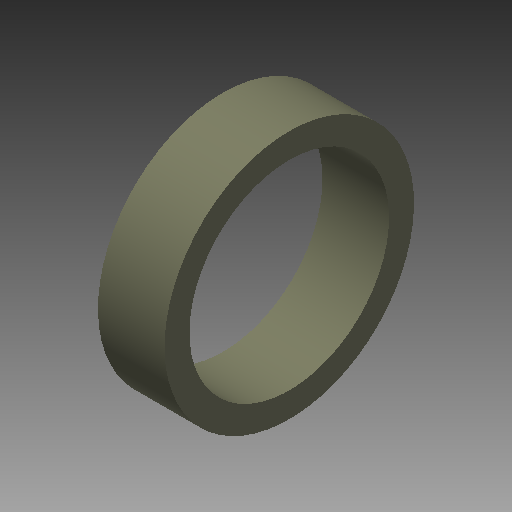
# Autodesk Inventor part: UMHSL30_k
Saved by Autodesk Inventor 2019 (Build 230136000, 136)
## iProperties
Category: PARTsolutions
Company: MISUMI
Created: 2015-12-01
Part Number: UMHSL30_k
Catalog Web Link: www.cadenas.de
Description: UMHSH, UMHS, UMHSL ,UMHAH, UMHA, UMHAL_k-Urethane Rollers - Set Screw Type
Vendor: MISUMI
Document SubType Name: Modeling
Designer: psAdmin
Manufacturer: MISUMI
Mass: 2.03575 g
Surface Area: 18.6611 cm^2
Volume: 2.03575 cm^3
Density: 1 g/cm^3
Material: Generic
Appearance: PSOLRGB-252-255-188
PSOL_IDENT_0: {$CADENAS_DATA\23d-libs\misumi\metric\53_rollers\umhsh\umhsh_k.prj},201 {VTYP=3D},{NB=UMHSL30_k},{LI
PSOL_IDENT_1: NA=UMHSL30},{NN=UMHSH, UMHS, UMHSL ,UMHAH, UMHA, UMHAL_k},{DATE=06.11.2015 05:15:16},{GEOMDATE=30.10
PSOL_IDENT_2: .2015 01:03:12},{VERSION=},{LINEID=70},{LINESUBID=-1},{WBVAR=MATC,HARD}  {NB=UMHSL30_k},{LINA=UMHSL3
PSOL_IDENT_3: 0},{KT=DUMMY},{PN=UMHSL30},{TYPE=UMHSL},{MATC=1},{MATCALG= '1','304 Stainless Steel','2','5052 Alumi
PSOL_IDENT_4: num Alloy'},{MATU=Urethane (Natural Color)},{HARD=A50},{COLOR=0.99,1.00,0.74,0.00},{NO=30},{D=30},{D
PSOL_IDENT_5: D=6},{D1=16},{D2=24},{D2X=24},{W=8},{L=20},{R=6.0},{M=3}
NN: UMHSH, UMHS, UMHSL ,UMHAH, UMHA, UMHAL_k
NT: Urethane Rollers - Set Screw Type
NB: UMHSL30_k
NBSYN: $PN._k
LINA: UMHSL30
PN: UMHSL30
MATC: 304 Stainless Steel
MATU: Urethane (Natural Color)
HARD: Shore A50
NO: 30
D: 30
DD: 6
D1: 16
D2: 24
W: 8
L: 20
M: 3
SUPPLIER: MISUMI
ARTICLENO: UMHSL30_k
BOMINFO: UMHSL30
CREATOR: CADENAS GmbH
Title: UMHSL30
Author: Cadenas PARTsolutions
Comments: Urethane Rollers - Set Screw Type
Autodesk Inventor part; units mm, degrees
sketch "Sketch_1" plane through (0, 0, 0) normal (0, 0, 1) x (1, 0, 0)
  line L0 (4, 0) -> (-4, 0)
  line L1 (-4, 15) -> (-4, 12)
  line L2 (-4, 12) -> (4, 12)
  line L3 (4, 12) -> (4, 15)
  line L4 (4, 15) -> (-4, 15)
  constraints: 10 end point
revolve "Revolution1" add sketch "Sketch_1" angle 360 about axis through (4, 0, 0) along (1, 0, 0)
ref_plane "k_c_XY" through (0, 0, 0) normal (-1, 0, 0) x (0, 0, -1)
ref_plane "k_c_YZ" through (0, 0, 0) normal (0, 0, -1) x (0, -1, 0)
ref_plane "k_c_ZX" through (0, 0, 0) normal (0, -1, 0) x (-1, 0, 0)
body "Solid1"
